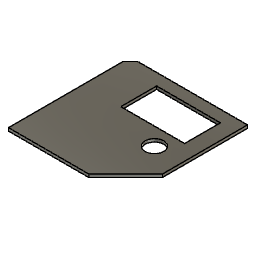
ECE198 Housing v1-5 (Autodesk Fusion 360 archive; units mm, degrees)
design "Lid"
Autodesk Fusion 360 part; units mm, degrees
other "DerivedContext1"
sketch "lid v2" plane through (-180, 0, 0) normal (0, 0, 1) x (1, 0, 0)
  line L0 (334.0338, -3.2613) -> (192.2917, -3.2613)
  line L1 (316.9875, -15.8281) -> (316.9875, -64.0063)
  line L2 (287.0338, -159.4636) -> (334.0338, -112.4636)
  line L3 (231.1593, -15.8281) -> (316.9875, -15.8281)
  line L4 (337.6529, -114.5635) -> (288.1529, -164.0635)
  line L5 (192.2917, -3.2613) -> (183.2917, -12.2613)
  line L6 (334.0338, -112.4636) -> (334.0338, -3.2613)
  line L7 (183.2917, -12.2613) -> (183.2917, -159.4636)
  line L8 (316.9875, -64.0063) -> (231.1593, -64.0063)
  line L9 (183.2917, -159.4636) -> (287.0338, -159.4636)
  line L10 (180, -164.0635) -> (180, -10.5)
  line L11 (288.1529, -164.0635) -> (180, -164.0635)
  line L12 (180, -10.5) -> (190.5, 0)
  line L13 (337.6529, 0) -> (337.6529, -114.5635)
  line L14 (190.5, 0) -> (337.6529, 0)
  circle A0 centre (299.8198, -87.3938) radius 12.5
  line L15 (231.1593, -64.0063) -> (231.1593, -15.8281)
extrude "Extrude3" add sketch "lid v2" along normal blind 4 contours L0 L2 L5 L6 L7 L9 | L4 L10 L11 L12 L13 L14
